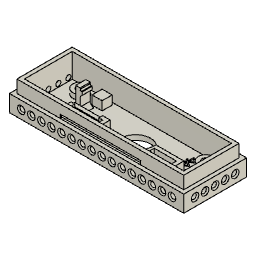
Outer Case Side Base v59 (Autodesk Fusion 360 design; units mm, degrees)
Autodesk Fusion 360 part; units mm, degrees
(part 1 of 2)
sketch "Sketch1" plane through (0, 0, 0) normal (0, 0, 1) x (1, 0, 0)
  line L0 (0, 0) -> (69.4, 0)
  line L1 (69.4, 0) -> (69.4, 25)
  line L2 (69.4, 25) -> (0, 25)
  line L3 (0, 25) -> (0, 0)
  line L4 (3, 3) -> (66.4, 3)
  line L5 (66.4, 3) -> (66.4, 22)
  line L6 (66.4, 22) -> (3, 22)
  line L7 (3, 22) -> (3, 3)
  circle A0 centre (9.7, 18.5) radius 3
  circle A1 centre (59.7, 18.5) radius 3
  circle A2 centre (9.7, 6.5) radius 3
  circle A3 centre (59.7, 6.5) radius 3
  circle A4 centre (9.7, 18.5) radius 1.5
  circle A5 centre (9.7, 6.5) radius 1.5
  circle A6 centre (59.7, 18.5) radius 1.5
  circle A7 centre (59.7, 6.5) radius 1.5
  dimension "d1" = 69.4
  dimension "d2" = 25
  dimension "d3" = -3
  dimension "d8" = 6
  dimension "d9" = 6
  dimension "d10" = 6
  dimension "d11" = 6
  dimension "d12" = 50
  dimension "d13" = 9.7
  dimension "d14" = 12
  dimension "d15" = 6.5
  dimension "d16" = 3
  dimension "d17" = 3
  dimension "d18" = 3
  dimension "d19" = 3
  dimension "d89" = 6.5
  constraint horizontal L0
  constraint vertical L1
  constraint horizontal L2
  constraint vertical L3
  constraint coincident L0.start L3.end
  constraint horizontal A0.centre A1.centre
  constraint horizontal A2.centre A3.centre
  constraint vertical A0.centre A2.centre
  constraint vertical A1.centre A3.centre
  constraint concentric A0 A4
  constraint concentric A2 A5
  constraint concentric A1 A6
  constraint concentric A3 A7
  measures "d1" distance of L0.start L0.end
  measures "d2" distance of L0.start L2.end
  measures "d8" diameter of A0
  measures "d9" diameter of A1
  measures "d10" diameter of A2
  measures "d11" diameter of A3
  measures "d12" distance of A0.centre A1.centre
  measures "d13" distance of L3 A0.centre
  measures "d14" distance of A0.centre A2.centre
  measures "d15" distance of L2 A0.centre
  measures "d16" diameter of A4
  measures "d17" diameter of A5
  measures "d18" diameter of A6
  measures "d19" diameter of A7
  measures "d89" distance of L0 A2.centre
extrude "Extrude3" add sketch "Sketch1" along normal blind 4 contours A0 | A1 | A2 | A3 makes body 1 at (12.6963, 6.3505, 2.6667) makes body 2 at (62.6963, 18.3505, 2.6667) makes body 3 at (12.6963, 18.3505, 2.6667) makes body 4 at (62.6963, 6.3505, 2.6667)
extrude "Extrude2" add sketch "Sketch1" along normal blind 2 contours L4 L5 L6 L7 | A0 | A1 | A2 | A3 bodies 1 2 3 4
extrude "Extrude1" add sketch "Sketch1" along normal blind 11.6 contours L0 L1 L2 L3 bodies 1
sketch "Sketch2" plane through (0, 0, 11.6) normal (0, 0, 1) x (-1, 0, 0)
  line L0 (-3, -3) -> (-3, -22)
  line L1 (-3, -22) -> (-66.4, -22)
  line L2 (-66.4, -22) -> (-66.4, -3)
  line L3 (-66.4, -3) -> (-3, -3)
  line L4 (0, -25) -> (0, 0)
  line L5 (0, 0) -> (-69.4, 0)
  line L6 (-69.4, 0) -> (-69.4, -25)
  line L7 (-69.4, -25) -> (0, -25)
  line L8 (-1.5, -1.5) -> (-67.9, -1.5)
  line L9 (-67.9, -1.5) -> (-67.9, -23.5)
  line L10 (-67.9, -23.5) -> (-1.5, -23.5)
  line L11 (-1.5, -23.5) -> (-1.5, -1.5)
  dimension "d22" = -1.5
extrude "Extrude4" cut sketch "Sketch2" against normal blind 5 contours L4 L5 L6 L7 bodies 1
sketch "Sketch3" plane through (0, 0, 2) normal (0, 0, 1) x (-1, 0, 0)
  line L0 (-15.5, -10.5) -> (-26.6, -10.5)
  line L1 (-26.6, -10.5) -> (-26.6, -7.8)
  line L2 (-26.6, -7.8) -> (-15.5, -7.8)
  line L3 (-15.5, -7.8) -> (-15.5, -10.5)
  line L4 (-28.1, -6.3) -> (-14, -6.3)
  line L5 (-14, -6.3) -> (-14, -12)
  line L6 (-14, -12) -> (-28.1, -12)
  line L7 (-28.1, -12) -> (-28.1, -6.3)
  line L8 (-47.6, -10.05) -> (-56.4, -10.05)
  line L9 (-56.4, -10.05) -> (-56.4, -6)
  line L10 (-56.4, -6) -> (-47.6, -6)
  line L11 (-47.6, -6) -> (-47.6, -10.05)
  line L12 (-3, -22) -> (-3, -3)
  line L13 (-57.9, -4.5) -> (-46.1, -4.5)
  line L14 (-46.1, -4.5) -> (-46.1, -11.55)
  line L15 (-46.1, -11.55) -> (-57.9, -11.55)
  line L16 (-57.9, -11.55) -> (-57.9, -4.5)
  line L17 (-13.7613, -3.1356) -> (-28.6187, -3.1356) construction
  line L18 (-28.6187, -3.1356) -> (-28.6187, -7.1356) construction
  line L19 (-28.6187, -7.1356) -> (-13.7613, -7.1356) construction
  line L20 (-13.7613, -7.1356) -> (-13.7613, -3.1356) construction
  line L21 (-47.2804, -11.8748) -> (-52.7589, -11.8748) construction
  line L22 (-52.7589, -11.8748) -> (-52.7589, -15.8748) construction
  line L23 (-52.7589, -15.8748) -> (-47.2804, -15.8748) construction
  line L24 (-47.2804, -15.8748) -> (-47.2804, -11.8748) construction
  line L25 (-56.651, -11.8238) -> (-64.2721, -11.8238) construction
  line L26 (-64.2721, -11.8238) -> (-64.2721, -15.8238) construction
  line L27 (-64.2721, -15.8238) -> (-56.651, -15.8238) construction
  line L28 (-56.651, -15.8238) -> (-56.651, -11.8238) construction
  line L29 (-15.85, -21.05) -> (-19.85, -21.05)
  line L30 (-19.85, -21.05) -> (-19.85, -17.05)
  line L31 (-19.85, -17.05) -> (-15.85, -17.05)
  line L32 (-15.85, -17.05) -> (-15.85, -21.05)
  line L33 (-15.65, -16.5) -> (-13.9, -16.5)
  line L34 (-13.9, -16.5) -> (-13.9, -12.5)
  line L35 (-13.9, -12.5) -> (-15.65, -12.5)
  line L36 (-15.65, -12.5) -> (-15.65, -16.5)
  circle A0 centre (-59.7, -6.5) radius 3
  circle A1 centre (-9.7, -18.5) radius 3
  circle A2 centre (-59.7, -18.5) radius 3
  circle A3 centre (-9.7, -6.5) radius 3
  line L37 (-3, -22) -> (-3, -3)
  line L38 (-3, -3) -> (-66.4, -3)
  line L39 (-66.4, -3) -> (-66.4, -22)
  line L40 (-66.4, -22) -> (-3, -22)
  circle A4 centre (-38.9, -11.38) radius 5.9
  circle A5 centre (-38.9, -11.38) radius 7.375
  line L41 (-44, -14.3465) -> (-44, -8.4135)
  line L42 (-69.4, 0) -> (0, 0)
  line L43 (-69.4, -25) -> (-69.4, 0)
  dimension "d25" = 2.7
  dimension "d26" = 11.1
  dimension "d27" = -1.5
  dimension "d32" = 8.8
  dimension "d33" = 4.05
  dimension "d36" = 11
  dimension "d70" = -1.5
  dimension "d95" = 13.25
  dimension "d97" = 4
  dimension "d98" = 1.75
  dimension "d99" = 4
  dimension "d100" = 4
  dimension "d126" = 4.8
  dimension "d127" = 10
  dimension "d128" = 3
  dimension "d129" = 11.8
  dimension "d133" = 7.2279
  dimension "d134" = 7.2
  dimension "d135" = 14.75
  dimension "d138" = 11.38
  dimension "d139" = 30.5
  dimension "d142" = 0.15
  dimension "d143" = 0.2
  dimension "d145" = 5.1
  text T0 "BMP280" font "Arial" height 4 align ink ink in box 0 x 0 at (-13.7613, -3.1356) x (-1, 0) y (0, -1) spacing 1 height is em
  text T1 "ON" font "Arial" height 4 align ink ink in box 0 x 0 at (-47.2804, -11.8748) x (-1, 0) y (0, -1) spacing 1 height is em
  text T2 "OFF" font "Arial" height 4 align ink ink in box 0 x 0 at (-56.651, -11.8238) x (-1, 0) y (0, -1) spacing 1 height is em
  constraint horizontal L0
  constraint vertical L1
  constraint horizontal L2
  constraint vertical L3
  constraint horizontal L8
  constraint vertical L9
  constraint horizontal L10
  constraint vertical L11
  constraint perpendicular L17 L18
  constraint parallel L17 L19
  constraint parallel L18 L20
  constraint perpendicular L21 L22
  constraint parallel L21 L23
  constraint parallel L22 L24
  constraint perpendicular L25 L26
  constraint parallel L25 L27
  constraint parallel L26 L28
  constraint horizontal L29
  constraint vertical L30
  constraint horizontal L31
  constraint vertical L32
  constraint horizontal L33
  constraint vertical L34
  constraint horizontal L35
  constraint vertical L36
  constraint coincident L31.end L32.start
  constraint coincident L33.start L36.end
  constraint concentric A4 A5
  constraint coincident A4 L41.start
  constraint coincident A4 L41.end
  constraint perpendicular L40 L41
  constraint horizontal L21
  constraint horizontal L25
  measures "d25" distance of L0.start L2.end
  measures "d26" distance of L0.start L0.end
  measures "d32" distance of L8.start L8.end
  measures "d33" distance of L8.start L10.end
  measures "d36" distance of L5 L12
  measures "d95" distance of L2 L29
  measures "d97" distance of L29.end L30.end
  measures "d98" distance of L33.start L33.end
  measures "d99" distance of L33.start L35.end
  measures "d100" distance of L29.start L29.end
  measures "d126" distance of L2 L38
  measures "d127" distance of L9 L39
  measures "d128" distance of L10 L38
  measures "d129" diameter of A4
  measures "d134" distance of L14 A4.centre
  measures "d135" diameter of A5
  measures "d138" distance of A4.centre L42
  measures "d139" distance of A4.centre L43
  measures "d142" distance of L3 L36
  measures "d143" distance of L32 L36
  measures "d145" distance of A4.centre L41
extrude "Extrude19" [suppressed]
extrude "Extrude18" cut sketch "Sketch3" against normal blind 4 contours A4 L41 picked at (-40.3333, -11.38) bodies 1
extrude "Extrude16" add sketch "Sketch3" along normal blind 5.1 contours L33 L34 L35 L36 bodies 1
extrude "Extrude14" cut sketch "Sketch3" against normal blind 0.5 text T1 T2 T0 bodies 1
extrude "Extrude11" add sketch "Sketch3" along normal blind 4.5 contours L13 L16 A0 | L13 L14 L15 L16 A0 A5 | L14 L15 A5 picked at (-57.7996, -7.3471) picked at (-46.212, -11.3523) bodies 1
extrude "Extrude7" cut sketch "Sketch3" against normal blind 3 contours L8 L9 L10 L11 bodies 1
extrude "Extrude6" cut sketch "Sketch3" against normal blind 3 contours L0 L1 L2 L3 bodies 1
extrude "Extrude5" add sketch "Sketch3" along normal blind 3.5 contours L4 L5 L6 L7 | L29 L30 L31 L32 bodies 1
sketch "Sketch4" plane through (0, 0, 0) normal (-1, 0, 0) x (0, -1, 0)
  line L0 (0, 6.6) -> (-25, 6.6)
  line L1 (-25, 6.6) -> (-25, 0)
  line L2 (-25, 0) -> (0, 0)
  line L3 (0, 0) -> (0, 6.6)
  circle A0 centre (-20.5, 3.3) radius 1
  circle A1 centre (-16.5, 3.3) radius 1
  circle A2 centre (-12.5, 3.3) radius 1
  circle A3 centre (-8.5, 3.3) radius 1
  circle A4 centre (-4.5, 3.3) radius 1
  line L4 (-25, 0) -> (0, 0)
  dimension "d40" = 2
  dimension "d43" = 4
  dimension "d44" = 0
  dimension "d47" = 3.3
  dimension "d48" = 4.5
  dimension "d68" = 25
  measures "d40" diameter of A0
  measures "d47" distance of A0.centre L4
  measures "d48" distance of L1 A0.centre
  measures "d68" distance of L1.end L2.end
extrude "Extrude8" cut sketch "Sketch4" against normal blind 3.1 contours A0 | A1 | A2 | A3 | A4 bodies 1
sketch "Sketch5" plane through (69.4, 0, 0) normal (1, 0, 0) x (0, 1, 0)
  line L0 (25, 6.6) -> (0, 6.6)
  line L1 (0, 6.6) -> (0, 0)
  line L2 (0, 0) -> (25, 0)
  line L3 (25, 0) -> (25, 6.6)
  circle A0 centre (4.5, 3.3) radius 1
  circle A1 centre (8.5, 3.3) radius 1
  circle A2 centre (12.5, 3.3) radius 1
  circle A3 centre (16.5, 3.3) radius 1
  circle A4 centre (20.5, 3.3) radius 1
  line L4 (0, 0) -> (25, 0)
  dimension "d49" = 2
  dimension "d52" = 4
  dimension "d53" = 0
  dimension "d54" = 3.3
  dimension "d55" = 4.5
  dimension "d69" = 25
  measures "d49" diameter of A0
  measures "d54" distance of A4.centre L4
  measures "d55" distance of L3 A4.centre
  measures "d69" distance of L1.end L2.end
extrude "Extrude9" cut sketch "Sketch5" against normal blind 3.1 contours A0 | A1 | A2 | A3 | A4 bodies 1
sketch "Sketch6" plane through (0, 0, 0) normal (0, -1, 0) x (1, 0, 0)
  line L0 (69.4, 6.6) -> (0, 6.6)
  line L1 (0, 6.6) -> (0, 0)
  line L2 (0, 0) -> (69.4, 0)
  line L3 (69.4, 0) -> (69.4, 6.6)
  circle A0 centre (4.7, 3.3) radius 1
  circle A1 centre (8.7, 3.3) radius 1
  circle A2 centre (12.7, 3.3) radius 1
  circle A3 centre (16.7, 3.3) radius 1
  circle A4 centre (20.7, 3.3) radius 1
  circle A5 centre (24.7, 3.3) radius 1
  circle A6 centre (28.7, 3.3) radius 1
  circle A7 centre (32.7, 3.3) radius 1
  circle A8 centre (36.7, 3.3) radius 1
  circle A9 centre (40.7, 3.3) radius 1
  circle A10 centre (44.7, 3.3) radius 1
  circle A11 centre (48.7, 3.3) radius 1
  circle A12 centre (52.7, 3.3) radius 1
  circle A13 centre (56.7, 3.3) radius 1
  circle A14 centre (60.7, 3.3) radius 1
  circle A15 centre (64.7, 3.3) radius 1
  line L4 (0, 0) -> (69.4, 0)
  dimension "d58" = 2
  dimension "d61" = 4
  dimension "d62" = 0
  dimension "d63" = 69.4
  dimension "d64" = 4.7
  dimension "d65" = 3.3
  measures "d58" diameter of A0
  measures "d63" distance of L1.end L2.end
  measures "d64" distance of L1 A0.centre
  measures "d65" distance of A0.centre L4
extrude "Extrude10" cut sketch "Sketch6" against normal blind 3 contours A0 | A1 | A2 | A3 | A4 | A5 | A6 | A7 | A8 | A9 | A10 | A11 | A12 | A13 | A14 | A15 bodies 1
chamfer "Chamfer3" distance 0.5 angle 45 26 edges at (69.4, 19.5677, 3.6616) (69.4, 15.5677, 3.6616) (69.4, 11.5677, 3.6616) (69.4, 7.5677, 3.6616) (69.4, 3.5677, 3.6616) (63.7677, 0, 3.6616) (59.7677, 0, 3.6616) (55.7677, 0, 3.6616) (51.7677, 0, 3.6616) (47.7677, 0, 3.6616) (43.7677, 0, 3.6616) (39.7677, 0, 3.6616) (35.7677, 0, 3.6616) (31.7677, 0, 3.6616) (27.7677, 0, 3.6616) (23.7677, 0, 3.6616) (19.7677, 0, 3.6616) (15.7677, 0, 3.6616) (11.7677, 0, 3.6616) (7.7677, 0, 3.6616) (3.7677, 0, 3.6616) (0, 5.4323, 3.6616) (0, 9.4323, 3.6616) (0, 13.4323, 3.6616) (0, 17.4323, 3.6616) (0, 21.4323, 3.6616) measured on face at (69.4, 23.8333, 3.3) measured on face at (69.4, 23.8333, 3.3) measured on face at (69.4, 23.8333, 3.3) measured on face at (69.4, 23.8333, 3.3) measured on face at (69.4, 23.8333, 3.3) measured on face at (1.2333, 0, 3.3) measured on face at (1.2333, 0, 3.3) measured on face at (1.2333, 0, 3.3) measured on face at (1.2333, 0, 3.3) measured on face at (1.2333, 0, 3.3) measured on face at (1.2333, 0, 3.3) measured on face at (1.2333, 0, 3.3) measured on face at (1.2333, 0, 3.3) measured on face at (1.2333, 0, 3.3) measured on face at (1.2333, 0, 3.3) measured on face at (1.2333, 0, 3.3) measured on face at (1.2333, 0, 3.3) measured on face at (1.2333, 0, 3.3) measured on face at (1.2333, 0, 3.3) measured on face at (1.2333, 0, 3.3) measured on face at (1.2333, 0, 3.3) measured on face at (0, 1.1667, 3.3) measured on face at (0, 1.1667, 3.3) measured on face at (0, 1.1667, 3.3) measured on face at (0, 1.1667, 3.3) measured on face at (0, 1.1667, 3.3) on bodies 1
sketch "Sketch9" plane through (0, 0, 7.1) normal (0, 0, 1) x (-1, 0, 0)
  line L0 (-15.65, -12.5) -> (-15.65, -16.5)
  line L1 (-15.65, -16.5) -> (-13.9, -16.5)
  line L2 (-13.9, -16.5) -> (-13.9, -12.5)
  line L3 (-13.9, -12.5) -> (-15.65, -12.5)
  line L4 (-13.9, -16.5) -> (-16.45, -16.5)
  line L5 (-16.45, -16.5) -> (-16.45, -12.5)
  line L6 (-16.45, -12.5) -> (-13.9, -12.5)
  line L7 (-13.9, -12.5) -> (-13.9, -16.5)
  dimension "d110" = 2.55
  constraint horizontal L4
  constraint vertical L5
  constraint horizontal L6
  constraint vertical L7
  constraint coincident L1.end L2.start
  measures "d110" distance of L1.end L4.end
extrude "Extrude17" add sketch "Sketch9" along normal blind 2 bodies 1
chamfer "Chamfer5" distance 0.8 angle 45 1 edges at (16.45, 14.5, 7.1) measured on face at (16.1833, 13.8333, 7.1) on bodies 1
sketch "Sketch10" plane through (0, 1.5, 0) normal (0, -1, 0) x (1, 0, 0)
  line L0 (67.9, 11.6) -> (1.5, 11.6)
  line L1 (1.5, 11.6) -> (1.5, 6.6)
  line L2 (1.5, 6.6) -> (67.9, 6.6)
  line L3 (67.9, 6.6) -> (67.9, 11.6)
  line L4 (18.7, 6.6) -> (50.7, 6.6)
  line L5 (50.7, 6.6) -> (50.7, 8.1)
  line L6 (50.7, 8.1) -> (18.7, 8.1)
  line L7 (18.7, 8.1) -> (18.7, 6.6)
  dimension "d115" = 32
  dimension "d116" = 1.5
  dimension "d117" = 66.4
  dimension "d118" = 17.2
  constraint horizontal L4
  constraint vertical L5
  constraint horizontal L6
  constraint vertical L7
  constraint coincident L2 L4.start
  measures "d115" distance of L4.start L4.end
  measures "d116" distance of L4.start L6.end
  measures "d117" distance of L0.start L0.end
  measures "d118" distance of L3 L5
revolve "Revolve1" cut sketch "Sketch10" angle 25 about axis through (50.7, 1.5, 8.1) along (1, 0, 0) contours L2 L4 L5 L6 L7 bodies 1
sketch "Sketch11" plane through (0, 23.5, 0) normal (0, 1, 0) x (-1, 0, 0)
  line L0 (-1.5, 11.6) -> (-67.9, 11.6)
  line L1 (-67.9, 11.6) -> (-67.9, 6.6)
  line L2 (-67.9, 6.6) -> (-1.5, 6.6)
  line L3 (-1.5, 6.6) -> (-1.5, 11.6)
  line L4 (-50.7, 6.6) -> (-18.7, 6.6)
  line L5 (-18.7, 6.6) -> (-18.7, 8.1)
  line L6 (-18.7, 8.1) -> (-50.7, 8.1)
  line L7 (-50.7, 8.1) -> (-50.7, 6.6)
  dimension "d120" = 32
  dimension "d121" = 1.5
  dimension "d122" = 66.4
  dimension "d123" = 17.2
  constraint horizontal L4
  constraint vertical L5
  constraint horizontal L6
  constraint vertical L7
  constraint coincident L2 L4.start
  measures "d120" distance of L4.start L4.end
  measures "d121" distance of L4.start L6.end
  measures "d122" distance of L0.start L0.end
  measures "d123" distance of L3 L5
revolve "Revolve2" cut sketch "Sketch11" angle 25 about axis through (18.7, 23.5, 8.1) along (-1, 0, 0) contours L2 L4 L5 L6 L7 bodies 1
sketch "Sketch12" plane through (0, 0, 2) normal (0, 0, 1) x (-1, 0, 0)
  line L0 (-15.85, -17.05) -> (-15.85, -21.05)
  line L1 (-15.85, -21.05) -> (-19.85, -21.05)
  line L2 (-19.85, -21.05) -> (-19.85, -17.05)
  line L3 (-19.85, -17.05) -> (-15.85, -17.05)
  line L4 (-28.1, -12) -> (-28.1, -6.3)
  line L5 (-28.1, -6.3) -> (-14, -6.3)
  line L6 (-14, -6.3) -> (-14, -12)
  line L7 (-14, -12) -> (-28.1, -12)
  line L8 (-57.9, -11.55) -> (-57.9, -8.9)
  arc A0 (-57.4639, -4.5) -> (-57.9, -8.9) centre (-59.7, -6.5) ccw
  line L9 (-57.4639, -4.5) -> (-46.1, -4.5)
  line L10 (-46.1, -4.5) -> (-46.1, -11.55)
  line L11 (-46.1, -11.55) -> (-57.9, -11.55)
  line L12 (-16.8084, -5.642) -> (-16.8084, -3.2045)
  line L13 (-16.8084, -3.2045) -> (-16.4431, -3.2045)
  line L14 (-16.4431, -3.2045) -> (-16.4431, -6.0678)
  line L15 (-16.4431, -6.0678) -> (-17.0134, -6.0678)
  line L16 (-17.0134, -6.0678) -> (-17.6912, -4.0404)
  spline S0 degree 3 poles (-17.6912, -4.0404) (-17.7185, -3.958) (-17.7651, -3.817) (-17.8095, -3.6754) (-17.8279, -3.6166) knots 0 0 0 0 0.026049 0.044534 0.044534 0.044534 0.044534
  spline S1 degree 3 poles (-17.8279, -3.6166) (-17.8486, -3.6809) (-17.8979, -3.8344) (-17.95, -3.987) (-17.9802, -4.0756) knots 0 0 0 0 0.020274 0.048362 0.048362 0.048362 0.048362
  line L17 (-17.9802, -4.0756) -> (-18.6658, -6.0678)
  line L18 (-18.6658, -6.0678) -> (-19.1756, -6.0678)
  line L19 (-19.1756, -6.0678) -> (-19.1756, -3.2045)
  line L20 (-19.1756, -3.2045) -> (-18.8103, -3.2045)
  line L21 (-18.8103, -3.2045) -> (-18.8103, -5.601)
  line L22 (-18.8103, -5.601) -> (-17.9783, -3.2045)
  line L23 (-17.9783, -3.2045) -> (-17.6365, -3.2045)
  line L24 (-17.6365, -3.2045) -> (-16.8084, -5.642)
  spline S2 degree 3 poles (-27.6951, -3.1556) (-27.5655, -3.1667) (-27.3128, -3.1883) (-27.1326, -3.3659) (-27.0447, -3.4525) knots 0 0 0 0 0.037701 0.073534 0.073534 0.073534 0.073534
  spline S3 degree 3 poles (-27.0447, -3.4525) (-26.9626, -3.606) (-26.7692, -3.9674) (-26.7643, -4.3795) (-26.7615, -4.6166) knots 0 0 0 0 0.051552 0.121345 0.121345 0.121345 0.121345
  spline S4 degree 3 poles (-26.7615, -4.6166) (-26.7636, -4.7702) (-26.7673, -5.047) (-26.8356, -5.3148) (-26.866, -5.434) knots 0 0 0 0 0.0459 0.082658 0.082658 0.082658 0.082658
  spline S5 degree 3 poles (-26.866, -5.434) (-26.903, -5.5295) (-26.9732, -5.7107) (-27.1113, -5.8471) (-27.1765, -5.9115) knots 0 0 0 0 0.030338 0.057541 0.057541 0.057541 0.057541
  spline S6 degree 3 poles (-27.1765, -5.9115) (-27.2518, -5.9605) (-27.4092, -6.0629) (-27.597, -6.0738) (-27.6951, -6.0795) knots 0 0 0 0 0.026458 0.055354 0.055354 0.055354 0.055354
  spline S7 degree 3 poles (-27.6951, -6.0795) (-27.7683, -6.0763) (-27.9088, -6.0701) (-28.0376, -6.0137) (-28.0994, -5.9867) knots 0 0 0 0 0.021755 0.0418 0.0418 0.0418 0.0418
  spline S8 degree 3 poles (-28.0994, -5.9867) (-28.1551, -5.9519) (-28.2681, -5.8814) (-28.3466, -5.7737) (-28.3865, -5.7191) knots 0 0 0 0 0.019498 0.039572 0.039572 0.039572 0.039572
  spline S9 degree 3 poles (-28.3865, -5.7191) (-28.4227, -5.6556) (-28.4995, -5.5211) (-28.5419, -5.372) (-28.5642, -5.2933) knots 0 0 0 0 0.021862 0.046289 0.046289 0.046289 0.046289
  spline S10 degree 3 poles (-28.5642, -5.2933) (-28.583, -5.1954) (-28.6257, -4.972) (-28.6276, -4.7444) (-28.6287, -4.6166) knots 0 0 0 0 0.029862 0.068104 0.068104 0.068104 0.068104
  spline S11 degree 3 poles (-28.6287, -4.6166) (-28.6266, -4.4639) (-28.6228, -4.1886) (-28.5553, -3.9219) (-28.5252, -3.8031) knots 0 0 0 0 0.045606 0.082253 0.082253 0.082253 0.082253
  spline S12 degree 3 poles (-28.5252, -3.8031) (-28.4884, -3.7075) (-28.4186, -3.526) (-28.2808, -3.3893) (-28.2156, -3.3246) knots 0 0 0 0 0.030329 0.05757 0.05757 0.05757 0.05757
  spline S13 degree 3 poles (-28.2156, -3.3246) (-28.1402, -3.2753) (-27.9823, -3.1722) (-27.7937, -3.1613) (-27.6951, -3.1556) knots 0 0 0 0 0.026536 0.05558 0.05558 0.05558 0.05558
  spline S14 degree 3 poles (-24.533, -4.0326) (-24.5377, -4.1203) (-24.5468, -4.2881) (-24.6333, -4.4318) (-24.6746, -4.5004) knots 0 0 0 0 0.025902 0.04954 0.04954 0.04954 0.04954
  spline S15 degree 3 poles (-24.6746, -4.5004) (-24.7283, -4.5586) (-24.8399, -4.6795) (-24.9966, -4.7307) (-25.0779, -4.7572) knots 0 0 0 0 0.023359 0.04853 0.04853 0.04853 0.04853
  spline S16 degree 3 poles (-25.0779, -4.7572) (-25.0111, -4.7849) (-24.8856, -4.8369) (-24.7957, -4.9383) (-24.7537, -4.9857) knots 0 0 0 0 0.021379 0.040128 0.040128 0.040128 0.040128
  spline S17 degree 3 poles (-24.7537, -4.9857) (-24.7229, -5.0388) (-24.6592, -5.1486) (-24.652, -5.2755) (-24.6482, -5.3412) knots 0 0 0 0 0.018126 0.037544 0.037544 0.037544 0.037544
  spline S18 degree 3 poles (-24.6482, -5.3412) (-24.6575, -5.4411) (-24.6759, -5.6404) (-24.8073, -5.7913) (-24.8728, -5.8666) knots 0 0 0 0 0.029303 0.058444 0.058444 0.058444 0.058444
  spline S19 degree 3 poles (-24.8728, -5.8666) (-24.9568, -5.9286) (-25.134, -6.0595) (-25.3545, -6.0726) (-25.4705, -6.0795) knots 0 0 0 0 0.030658 0.064671 0.064671 0.064671 0.064671
  spline S20 degree 3 poles (-25.4705, -6.0795) (-25.5873, -6.0723) (-25.8104, -6.0585) (-25.989, -5.9252) (-26.074, -5.8617) knots 0 0 0 0 0.034273 0.065414 0.065414 0.065414 0.065414
  spline S21 degree 3 poles (-26.074, -5.8617) (-26.1406, -5.7853) (-26.2736, -5.633) (-26.2929, -5.4317) (-26.3025, -5.3314) knots 0 0 0 0 0.02961 0.059051 0.059051 0.059051 0.059051
  spline S22 degree 3 poles (-26.3025, -5.3314) (-26.2986, -5.2679) (-26.2911, -5.144) (-26.2285, -5.0369) (-26.198, -4.9847) knots 0 0 0 0 0.01881 0.036662 0.036662 0.036662 0.036662
  spline S23 degree 3 poles (-26.198, -4.9847) (-26.1567, -4.9377) (-26.0687, -4.8375) (-25.9458, -4.785) (-25.8806, -4.7572) knots 0 0 0 0 0.018541 0.039496 0.039496 0.039496 0.039496
  spline S24 degree 3 poles (-25.8806, -4.7572) (-25.9622, -4.7257) (-26.1184, -4.6652) (-26.2291, -4.5398) (-26.282, -4.4799) knots 0 0 0 0 0.025791 0.049427 0.049427 0.049427 0.049427
  spline S25 degree 3 poles (-26.282, -4.4799) (-26.3222, -4.4116) (-26.4051, -4.2707) (-26.4147, -4.1072) (-26.4197, -4.0228) knots 0 0 0 0 0.023398 0.048344 0.048344 0.048344 0.048344
  spline S26 degree 3 poles (-26.4197, -4.0228) (-26.4091, -3.9055) (-26.388, -3.6722) (-26.2357, -3.4942) (-26.1599, -3.4056) knots 0 0 0 0 0.034407 0.068461 0.068461 0.068461 0.068461
  spline S27 degree 3 poles (-26.1599, -3.4056) (-26.0636, -3.3328) (-25.8618, -3.1801) (-25.6086, -3.164) (-25.4763, -3.1556) knots 0 0 0 0 0.035444 0.074232 0.074232 0.074232 0.074232
  spline S28 degree 3 poles (-25.4763, -3.1556) (-25.344, -3.1641) (-25.0907, -3.1803) (-24.8891, -3.3335) (-24.7927, -3.4066) knots 0 0 0 0 0.038792 0.074275 0.074275 0.074275 0.074275
  spline S29 degree 3 poles (-24.7927, -3.4066) (-24.717, -3.4961) (-24.5638, -3.677) (-24.5433, -3.9132) (-24.533, -4.0326) knots 0 0 0 0 0.034274 0.069281 0.069281 0.069281 0.069281
  line L25 (-62.7294, -13.1835) -> (-62.7294, -11.8827)
  line L26 (-62.7294, -11.8827) -> (-62.3505, -11.8827)
  line L27 (-62.3505, -11.8827) -> (-62.3505, -14.746)
  line L28 (-62.3505, -14.746) -> (-64.2821, -14.746)
  line L29 (-64.2821, -14.746) -> (-64.2821, -14.4081)
  line L30 (-64.2821, -14.4081) -> (-62.7294, -14.4081)
  line L31 (-62.7294, -14.4081) -> (-62.7294, -13.5213)
  line L32 (-62.7294, -13.5213) -> (-64.0731, -13.5213)
  line L33 (-64.0731, -13.5213) -> (-64.0731, -13.1835)
  line L34 (-64.0731, -13.1835) -> (-62.7294, -13.1835)
  line L35 (-50.8763, -14.1836) -> (-50.8763, -11.9336)
  line L36 (-50.8763, -11.9336) -> (-50.513, -11.9336)
  line L37 (-50.513, -11.9336) -> (-50.513, -14.7969)
  line L38 (-50.513, -14.7969) -> (-50.9017, -14.7969)
  line L39 (-50.9017, -14.7969) -> (-52.4056, -12.5488)
  line L40 (-52.4056, -12.5488) -> (-52.4056, -14.7969)
  line L41 (-52.4056, -14.7969) -> (-52.7689, -14.7969)
  line L42 (-52.7689, -14.7969) -> (-52.7689, -11.9336)
  line L43 (-52.7689, -11.9336) -> (-52.3802, -11.9336)
  line L44 (-52.3802, -11.9336) -> (-50.8763, -14.1836)
  spline S30 degree 3 poles (-47.9369, -12.0801) (-47.8371, -12.1512) (-47.6374, -12.2937) (-47.5155, -12.5067) (-47.4544, -12.6133) knots 0 0 0 0 0.03628 0.072668 0.072668 0.072668 0.072668
  spline S31 degree 3 poles (-47.2904, -13.3281) (-47.3014, -13.5474) (-47.3222, -13.9578) (-47.5617, -14.2898) (-47.6732, -14.4444) knots 0 0 0 0 0.064266 0.120259 0.120259 0.120259 0.120259
  spline S32 degree 3 poles (-47.6732, -14.4444) (-47.8124, -14.562) (-48.0977, -14.803) (-48.4705, -14.8325) (-48.6615, -14.8477) knots 0 0 0 0 0.053269 0.109167 0.109167 0.109167 0.109167
  spline S33 degree 3 poles (-48.6615, -14.8477) (-48.7894, -14.8404) (-49.0407, -14.826) (-49.2658, -14.7135) (-49.3763, -14.6582) knots 0 0 0 0 0.037992 0.074647 0.074647 0.074647 0.074647
  spline S34 degree 3 poles (-49.3763, -14.6582) (-49.4763, -14.5886) (-49.6772, -14.4485) (-49.8, -14.2365) (-49.8617, -14.1299) knots 0 0 0 0 0.036074 0.072525 0.072525 0.072525 0.072525
  spline S35 degree 3 poles (-49.8617, -14.1299) (-49.9103, -14.0109) (-50.0111, -13.7647) (-50.0227, -13.4988) (-50.0286, -13.3613) knots 0 0 0 0 0.038265 0.079177 0.079177 0.079177 0.079177
  spline S36 degree 3 poles (-50.0286, -13.3613) (-50.0223, -13.2219) (-50.01, -12.9515) (-49.9041, -12.7026) (-49.8529, -12.582) knots 0 0 0 0 0.041493 0.080461 0.080461 0.080461 0.080461
  spline S37 degree 3 poles (-49.8529, -12.582) (-49.7889, -12.4748) (-49.6626, -12.2632) (-49.4565, -12.1282) (-49.3548, -12.0615) knots 0 0 0 0 0.036922 0.072885 0.072885 0.072885 0.072885
  spline S38 degree 3 poles (-49.3548, -12.0615) (-49.245, -12.01) (-49.0246, -11.9065) (-48.7815, -11.892) (-48.6595, -11.8848) knots 0 0 0 0 0.036024 0.072329 0.072329 0.072329 0.072329
  spline S39 degree 3 poles (-48.6595, -11.8848) (-48.5295, -11.8922) (-48.2748, -11.9068) (-48.0479, -12.0231) (-47.9369, -12.0801) knots 0 0 0 0 0.038591 0.075598 0.075598 0.075598 0.075598
  line L45 (-60.286, -13.1835) -> (-60.286, -11.8827)
  line L46 (-60.286, -11.8827) -> (-59.9071, -11.8827)
  line L47 (-59.9071, -11.8827) -> (-59.9071, -14.746)
  line L48 (-59.9071, -14.746) -> (-61.8388, -14.746)
  line L49 (-61.8388, -14.746) -> (-61.8388, -14.4081)
  line L50 (-61.8388, -14.4081) -> (-60.286, -14.4081)
  line L51 (-60.286, -14.4081) -> (-60.286, -13.5213)
  line L52 (-60.286, -13.5213) -> (-61.6298, -13.5213)
  line L53 (-61.6298, -13.5213) -> (-61.6298, -13.1835)
  line L54 (-61.6298, -13.1835) -> (-60.286, -13.1835)
  spline S40 degree 3 poles (-57.3075, -12.0292) (-57.2078, -12.1003) (-57.008, -12.2428) (-56.8861, -12.4557) (-56.8251, -12.5624) knots 0 0 0 0 0.03628 0.072668 0.072668 0.072668 0.072668
  spline S41 degree 3 poles (-56.8251, -12.5624) (-56.7772, -12.6767) (-56.6814, -12.9055) (-56.6678, -13.1532) (-56.661, -13.2772) knots 0 0 0 0 0.036879 0.073826 0.073826 0.073826 0.073826
  spline S42 degree 3 poles (-56.661, -13.2772) (-56.6721, -13.4965) (-56.6928, -13.9068) (-56.9323, -14.2388) (-57.0438, -14.3934) knots 0 0 0 0 0.064266 0.120259 0.120259 0.120259 0.120259
  spline S43 degree 3 poles (-57.0438, -14.3934) (-57.183, -14.511) (-57.4683, -14.7521) (-57.8412, -14.7816) (-58.0321, -14.7967) knots 0 0 0 0 0.053269 0.109167 0.109167 0.109167 0.109167
  spline S44 degree 3 poles (-58.0321, -14.7967) (-58.16, -14.7894) (-58.4114, -14.7751) (-58.6364, -14.6625) (-58.747, -14.6073) knots 0 0 0 0 0.037992 0.074647 0.074647 0.074647 0.074647
  spline S45 degree 3 poles (-58.747, -14.6073) (-58.8469, -14.5376) (-59.0479, -14.3975) (-59.1706, -14.1855) (-59.2323, -14.079) knots 0 0 0 0 0.036074 0.072525 0.072525 0.072525 0.072525
  spline S46 degree 3 poles (-59.2323, -14.079) (-59.281, -13.96) (-59.3818, -13.7138) (-59.3933, -13.4478) (-59.3993, -13.3104) knots 0 0 0 0 0.038265 0.079177 0.079177 0.079177 0.079177
  spline S47 degree 3 poles (-59.3993, -13.3104) (-59.3929, -13.171) (-59.3806, -12.9006) (-59.2748, -12.6517) (-59.2235, -12.5311) knots 0 0 0 0 0.041493 0.080461 0.080461 0.080461 0.080461
  spline S48 degree 3 poles (-59.2235, -12.5311) (-59.1595, -12.4239) (-59.0333, -12.2122) (-58.8272, -12.0772) (-58.7255, -12.0106) knots 0 0 0 0 0.036922 0.072885 0.072885 0.072885 0.072885
  spline S49 degree 3 poles (-58.7255, -12.0106) (-58.6157, -11.959) (-58.3953, -11.8555) (-58.1522, -11.8411) (-58.0302, -11.8338) knots 0 0 0 0 0.036024 0.072329 0.072329 0.072329 0.072329
  spline S50 degree 3 poles (-58.0302, -11.8338) (-57.9001, -11.8413) (-57.6454, -11.8558) (-57.4186, -11.9722) (-57.3075, -12.0292) knots 0 0 0 0 0.038591 0.075598 0.075598 0.075598 0.075598
  spline S51 degree 3 poles (-22.9041, -3.7328) (-22.8758, -3.7018) (-22.8214, -3.6422) (-22.777, -3.5748) (-22.7556, -3.5424) knots 0 0 0 0 0.012549 0.024178 0.024178 0.024178 0.024178
  line L55 (-22.7556, -3.5424) -> (-24.1599, -3.5424)
  line L56 (-24.1599, -3.5424) -> (-24.1599, -3.2045)
  line L57 (-24.1599, -3.2045) -> (-22.2674, -3.2045)
  spline S52 degree 3 poles (-22.2674, -3.2045) (-22.2681, -3.2463) (-22.2695, -3.3298) (-22.2954, -3.4091) (-22.3084, -3.4486) knots 0 0 0 0 0.012479 0.024881 0.024881 0.024881 0.024881
  spline S53 degree 3 poles (-22.3084, -3.4486) (-22.3372, -3.5141) (-22.3975, -3.6512) (-22.491, -3.7683) (-22.5398, -3.8295) knots 0 0 0 0 0.021368 0.044735 0.044735 0.044735 0.044735
  spline S54 degree 3 poles (-22.5398, -3.8295) (-22.6034, -3.8982) (-22.7469, -4.0531) (-22.9094, -4.188) (-22.9998, -4.2631) knots 0 0 0 0 0.028058 0.063271 0.063271 0.063271 0.063271
  spline S55 degree 3 poles (-22.9998, -4.2631) (-23.1342, -4.3733) (-23.3607, -4.5589) (-23.5526, -4.7798) (-23.6306, -4.8695) knots 0 0 0 0 0.052022 0.087641 0.087641 0.087641 0.087641
  spline S56 degree 3 poles (-23.6306, -4.8695) (-23.6784, -4.9395) (-23.7661, -5.0682) (-23.7857, -5.2222) (-23.7947, -5.2924) knots 0 0 0 0 0.024992 0.04593 0.04593 0.04593 0.04593
  spline S57 degree 3 poles (-23.7947, -5.2924) (-23.7885, -5.3592) (-23.7762, -5.4927) (-23.6889, -5.5942) (-23.6453, -5.6449) knots 0 0 0 0 0.019622 0.039148 0.039148 0.039148 0.039148
  spline S58 degree 3 poles (-23.6453, -5.6449) (-23.5902, -5.6868) (-23.4752, -5.774) (-23.3308, -5.7835) (-23.2556, -5.7885) knots 0 0 0 0 0.020302 0.042349 0.042349 0.042349 0.042349
  spline S59 degree 3 poles (-23.2556, -5.7885) (-23.1765, -5.7834) (-23.0253, -5.7736) (-22.9062, -5.6805) (-22.8494, -5.6361) knots 0 0 0 0 0.023167 0.044296 0.044296 0.044296 0.044296
  spline S60 degree 3 poles (-22.8494, -5.6361) (-22.8049, -5.5779) (-22.71, -5.4538) (-22.7003, -5.2974) (-22.6951, -5.2142) knots 0 0 0 0 0.021485 0.045832 0.045832 0.045832 0.045832
  line L58 (-22.6951, -5.2142) -> (-22.3338, -5.2513)
  spline S61 degree 3 poles (-22.3338, -5.2513) (-22.3518, -5.3754) (-22.3857, -5.6086) (-22.5406, -5.785) (-22.6131, -5.8676) knots 0 0 0 0 0.0367 0.068958 0.068958 0.068958 0.068958
  spline S62 degree 3 poles (-22.6131, -5.8676) (-22.7047, -5.9293) (-22.9006, -6.0614) (-23.1374, -6.0732) (-23.2634, -6.0795) knots 0 0 0 0 0.032518 0.069569 0.069569 0.069569 0.069569
  spline S63 degree 3 poles (-23.2634, -6.0795) (-23.3909, -6.0725) (-23.6312, -6.0593) (-23.8248, -5.9175) (-23.9158, -5.851) knots 0 0 0 0 0.037354 0.070456 0.070456 0.070456 0.070456
  spline S64 degree 3 poles (-23.9158, -5.851) (-23.9859, -5.7699) (-24.1267, -5.607) (-24.1462, -5.3924) (-24.156, -5.2845) knots 0 0 0 0 0.031293 0.062923 0.062923 0.062923 0.062923
  spline S65 degree 3 poles (-24.156, -5.2845) (-24.153, -5.2272) (-24.1467, -5.111) (-24.1062, -5.0019) (-24.0857, -4.9467) knots 0 0 0 0 0.017131 0.03469 0.03469 0.03469 0.03469
  spline S66 degree 3 poles (-24.0857, -4.9467) (-24.0566, -4.8885) (-23.9933, -4.7624) (-23.9017, -4.655) (-23.8523, -4.597) knots 0 0 0 0 0.019438 0.042172 0.042172 0.042172 0.042172
  spline S67 degree 3 poles (-23.8523, -4.597) (-23.7809, -4.5234) (-23.609, -4.3462) (-23.4205, -4.1865) (-23.3103, -4.0931) knots 0 0 0 0 0.030746 0.074043 0.074043 0.074043 0.074043
  spline S68 degree 3 poles (-23.3103, -4.0931) (-23.2227, -4.02) (-23.0836, -3.904) (-22.9525, -3.779) (-22.9041, -3.7328) knots 0 0 0 0 0.034229 0.054317 0.054317 0.054317 0.054317
  line L59 (-20.1658, -4.3685) -> (-20.1658, -3.2045)
  line L60 (-20.1658, -3.2045) -> (-19.7869, -3.2045)
  line L61 (-19.7869, -3.2045) -> (-19.7869, -6.0678)
  line L62 (-19.7869, -6.0678) -> (-20.867, -6.0678)
  spline S69 degree 3 poles (-20.867, -6.0678) (-20.9509, -6.0675) (-21.0967, -6.067) (-21.2412, -6.0483) (-21.3025, -6.0404) knots 0 0 0 0 0.025156 0.043678 0.043678 0.043678 0.043678
  spline S70 degree 3 poles (-21.3025, -6.0404) (-21.3685, -6.027) (-21.4938, -6.0016) (-21.6039, -5.9371) (-21.656, -5.9066) knots 0 0 0 0 0.020045 0.038029 0.038029 0.038029 0.038029
  spline S71 degree 3 poles (-21.656, -5.9066) (-21.7017, -5.8695) (-21.7963, -5.7925) (-21.8551, -5.6856) (-21.8855, -5.6303) knots 0 0 0 0 0.017485 0.036225 0.036225 0.036225 0.036225
  spline S72 degree 3 poles (-21.8855, -5.6303) (-21.9109, -5.5689) (-21.9625, -5.4438) (-21.9691, -5.3085) (-21.9724, -5.2396) knots 0 0 0 0 0.019759 0.040284 0.040284 0.040284 0.040284
  spline S73 degree 3 poles (-21.9724, -5.2396) (-21.9634, -5.1233) (-21.9457, -4.8946) (-21.8078, -4.7115) (-21.74, -4.6215) knots 0 0 0 0 0.034213 0.067281 0.067281 0.067281 0.067281
  spline S74 degree 3 poles (-21.74, -4.6215) (-21.6347, -4.5481) (-21.3849, -4.3742) (-21.0778, -4.3706) (-20.9002, -4.3685) knots 0 0 0 0 0.037732 0.089487 0.089487 0.089487 0.089487
  line L63 (-20.9002, -4.3685) -> (-20.1658, -4.3685)
  spline S75 degree 3 poles (-15.325, -3.2523) (-15.2553, -3.2384) (-15.1029, -3.2079) (-14.9474, -3.2057) (-14.8631, -3.2045) knots 0 0 0 0 0.021277 0.046525 0.046525 0.046525 0.046525
  line L64 (-14.8631, -3.2045) -> (-13.7713, -3.2045)
  line L65 (-13.7713, -3.2045) -> (-13.7713, -6.0678)
  line L66 (-13.7713, -6.0678) -> (-14.8455, -6.0678)
  spline S76 degree 3 poles (-14.8455, -6.0678) (-14.945, -6.0659) (-15.125, -6.0626) (-15.2956, -6.0061) (-15.3718, -5.9808) knots 0 0 0 0 0.029645 0.05362 0.05362 0.05362 0.05362
  spline S77 degree 3 poles (-15.3718, -5.9808) (-15.4343, -5.9481) (-15.5585, -5.8829) (-15.6412, -5.7696) (-15.6824, -5.7133) knots 0 0 0 0 0.020838 0.041482 0.041482 0.041482 0.041482
  spline S78 degree 3 poles (-15.6824, -5.7133) (-15.7151, -5.653) (-15.7794, -5.5349) (-15.7897, -5.401) (-15.7947, -5.3353) knots 0 0 0 0 0.02031 0.039825 0.039825 0.039825 0.039825
  spline S79 degree 3 poles (-15.7947, -5.3353) (-15.7904, -5.2748) (-15.7817, -5.1525) (-15.7241, -5.0443) (-15.6951, -4.9896) knots 0 0 0 0 0.017995 0.036334 0.036334 0.036334 0.036334
  spline S80 degree 3 poles (-15.6951, -4.9896) (-15.6563, -4.9375) (-15.5752, -4.8286) (-15.4563, -4.7624) (-15.3943, -4.7279) knots 0 0 0 0 0.019257 0.040275 0.040275 0.040275 0.040275
  spline S81 degree 3 poles (-15.3943, -4.7279) (-15.4748, -4.6995) (-15.6291, -4.6449) (-15.7404, -4.5253) (-15.7937, -4.4681) knots 0 0 0 0 0.025178 0.048277 0.048277 0.048277 0.048277
  spline S82 degree 3 poles (-15.7937, -4.4681) (-15.8344, -4.4033) (-15.9177, -4.2707) (-15.9281, -4.1144) (-15.9334, -4.0345) knots 0 0 0 0 0.022594 0.046193 0.046193 0.046193 0.046193
  spline S83 degree 3 poles (-15.9334, -4.0345) (-15.93, -3.969) (-15.9233, -3.8394) (-15.8732, -3.7197) (-15.8484, -3.6605) knots 0 0 0 0 0.019525 0.038613 0.038613 0.038613 0.038613
  spline S84 degree 3 poles (-15.8484, -3.6605) (-15.8197, -3.6072) (-15.7652, -3.506) (-15.6791, -3.4299) (-15.6384, -3.3939) knots 0 0 0 0 0.018014 0.034173 0.034173 0.034173 0.034173
  spline S85 degree 3 poles (-15.6384, -3.3939) (-15.5925, -3.3642) (-15.4953, -3.3012) (-15.3838, -3.2692) (-15.325, -3.2523) knots 0 0 0 0 0.016314 0.034565 0.034565 0.034565 0.034565
  line L67 (-15.65, -12.5) -> (-13.9, -12.5)
  line L68 (-13.9, -12.5) -> (-13.9, -16.5)
  line L69 (-13.9, -16.5) -> (-15.65, -16.5)
  line L70 (-15.65, -16.5) -> (-15.65, -12.5)
  circle A1 centre (-9.7, -18.5) radius 3
  circle A2 centre (-59.7, -18.5) radius 3
  line L71 (-3, -22) -> (-3, -3)
  line L72 (-3, -3) -> (-66.4, -3)
  line L73 (-66.4, -3) -> (-66.4, -22)
  line L74 (-66.4, -22) -> (-3, -22)
  circle A3 centre (-9.7, -6.5) radius 3
  line L75 (-53.3471, -17.6537) -> (-54.2, -17)
  line L76 (-54.2, -17) -> (-54.2, -19.1)
  line L77 (-54.2, -19.1) -> (-54.7, -19.2)
  line L78 (-54.7, -19.2) -> (-56.3569, -17.93)
  line L79 (-56.3569, -17.93) -> (-56.3569, -17.6157)
  line L80 (-56.3569, -17.6157) -> (-54.8, -16.5)
  line L81 (-54.8, -16.5) -> (-56.2956, -15.447)
  line L82 (-56.2956, -15.447) -> (-56.2956, -15.2)
  line L83 (-56.2956, -15.2) -> (-54.5478, -13.8892)
  line L84 (-54.5478, -13.8892) -> (-54.3624, -13.8892)
  line L85 (-54.3624, -13.8892) -> (-54.1862, -14.0561)
  line L86 (-54.1862, -14.0561) -> (-54.1862, -16.0889)
  line L87 (-54.1862, -16.0889) -> (-53.3253, -15.472)
  line L88 (-53.3253, -15.472) -> (-53.0582, -15.8447)
  line L89 (-53.0582, -15.8447) -> (-54.0435, -16.5507)
  line L90 (-54.0435, -16.5507) -> (-53.0582, -17.32)
  line L91 (-53.0582, -17.32) -> (-53.3471, -17.6537)
  line L92 (-54.6684, -16.0889) -> (-55.7, -15.3)
  line L93 (-55.7, -15.3) -> (-54.6684, -14.5476)
  line L94 (-54.6684, -14.5476) -> (-54.6684, -16.0889)
  line L95 (-54.6684, -17.0001) -> (-55.7374, -17.7798)
  line L96 (-55.7374, -17.7798) -> (-54.6684, -18.5974)
  line L97 (-54.6684, -18.5974) -> (-54.6684, -17.0001)
  spline S86 degree 3 poles (-47.4544, -12.6133) (-47.4066, -12.7276) (-47.3108, -12.9565) (-47.2972, -13.2042) (-47.2904, -13.3281) knots 0 0 0 0 0.036879 0.073826 0.073826 0.073826 0.073826
  line L98 (-44, -14.3465) -> (-44, -8.4135)
  arc A4 (-44, -14.3465) -> (-44, -8.4135) centre (-38.9, -11.38) ccw
  constraint perpendicular L74 L76
  constraint parallel L75 L78
  constraint perpendicular L74 L79
  constraint perpendicular L74 L82
  constraint perpendicular L82 L84
  constraint perpendicular L84 L86
  constraint parallel L80 L87
  constraint perpendicular L80 L88
  constraint perpendicular L88 L89
  constraint vertical L94
  constraint parallel L93 L95
  constraint parallel L92 L96
  constraint parallel L94 L97
extrude "Extrude20" cut sketch "Sketch12" against normal blind 0.5 contours L75 L76 L77 L78 L79 L80 L81 L82 L83 L84 L85 L86 L87 L88 L89 L90 L91 bodies 1
fillet "Fillet2" radius 1.5 1 edges at (15.65, 14.5, 2) on bodies 1
sketch "Sketch20" plane through (0, 0, 5.5) normal (0, 0, 1) x (-1, 0, 0)
  line L0 (-26.6, -7.8) -> (-15.5, -7.8)
  line L1 (-15.5, -7.8) -> (-15.5, -10.5)
  line L2 (-15.5, -10.5) -> (-26.6, -10.5)
  line L3 (-26.6, -10.5) -> (-26.6, -7.8)
  line L4 (-28.1, -12) -> (-14, -12)
  line L5 (-14, -12) -> (-14, -6.3)
  line L6 (-14, -6.3) -> (-28.1, -6.3)
  line L7 (-28.1, -6.3) -> (-28.1, -12)
  line L8 (-25.1, -10.5) -> (-14, -10.5)
  line L9 (-14, -10.5) -> (-14, -12)
  line L10 (-14, -12) -> (-25.1, -12)
  line L11 (-25.1, -12) -> (-25.1, -10.5)
  line L12 (-28.1, -12) -> (-28.1, -6.3)
  dimension "d159" = 3
  constraint horizontal L8
  constraint vertical L9
  constraint horizontal L10
  constraint vertical L11
  constraint coincident L4.end L5.start
  constraint coincident L2 L8.start
  measures "d159" distance of L11 L12
extrude "Extrude24" cut sketch "Sketch20" against normal blind 1 contours L2 L4 L5 L8 L9 L10 L11 bodies 1